Autodesk Fusion 360 part; units mm, degrees
(part 2 of 4)
  spline S394 degree 3 poles (77.092, 15.6185) (76.8084, 15.0287) (76.6767, 14.3737) (76.5494, 13.7318) knots 0 0 0 0 1 1 1 1
  spline S395 degree 3 poles (76.5494, 13.7318) (76.4799, 13.3813) (76.5996, 13.0055) (76.5054, 12.6609) knots 0 0 0 0 1 1 1 1
  spline S396 degree 3 poles (76.5054, 12.6609) (76.401, 12.2788) (76.1059, 11.9726) (75.9671, 11.6017) knots 0 0 0 0 1 1 1 1
  spline S397 degree 3 poles (75.9671, 11.6017) (75.8459, 11.2776) (75.8098, 10.9278) (75.7312, 10.5909) knots 0 0 0 0 1 1 1 1
  spline S398 degree 3 poles (77.2579, 14.4353) (77.0942, 14.4652) (76.9305, 14.4951) (76.7668, 14.525) knots 0 0 0 0 1 1 1 1
  spline S399 degree 3 poles (76.2224, 10.5718) (76.0243, 10.4293) (75.7374, 10.3626) (75.6282, 10.1444) knots 0 0 0 0 1 1 1 1
  spline S400 degree 3 poles (75.6282, 10.1444) (75.4268, 9.7418) (75.3959, 9.2709) (75.3477, 8.8234) knots 0 0 0 0 1 1 1 1
  spline S401 degree 3 poles (75.3477, 8.8234) (75.2928, 8.3128) (75.3293, 7.7964) (75.3201, 7.2829) knots 0 0 0 0 1 1 1 1
  spline S402 degree 3 poles (74.77, 0.2181) (74.6504, 0.8429) (74.4776, 1.4598) (74.4114, 2.0925) knots 0 0 0 0 1 1 1 1
  spline S403 degree 3 poles (74.4114, 2.0925) (74.3786, 2.4055) (74.3986, 2.7292) (74.4753, 3.0344) knots 0 0 0 0 1 1 1 1
  spline S404 degree 3 poles (74.4753, 3.0344) (74.5407, 3.2944) (74.7115, 3.5157) (74.8296, 3.7563) knots 0 0 0 0 1 1 1 1
  spline S405 degree 3 poles (74.4084, 0.1917) (74.5689, 0.7067) (74.7884, 1.2069) (74.89, 1.7368) knots 0 0 0 0 1 1 1 1
  spline S406 degree 3 poles (74.89, 1.7368) (74.9706, 2.1572) (74.9634, 2.5918) (74.9506, 3.0197) knots 0 0 0 0 1 1 1 1
  spline S407 degree 3 poles (74.9506, 3.0197) (74.9432, 3.2684) (74.8081, 3.5084) (74.8296, 3.7563) knots 0 0 0 0 1 1 1 1
  spline S408 degree 3 poles (74.8296, 3.7563) (74.9321, 4.9387) (75.0884, 6.1189) (75.3201, 7.2829) knots 0 0 0 0 1 1 1 1
  spline S409 degree 3 poles (75.3201, 7.2829) (75.4212, 7.7908) (75.6863, 8.2533) (75.8241, 8.7525) knots 0 0 0 0 1 1 1 1
  spline S410 degree 3 poles (75.8241, 8.7525) (76.047, 9.5598) (76.2121, 10.382) (76.4009, 11.1979) knots 0 0 0 0 1 1 1 1
  spline S411 degree 3 poles (76.4009, 11.1979) (76.444, 11.3845) (76.5062, 11.569) (76.5199, 11.76) knots 0 0 0 0 1 1 1 1
  spline S412 degree 3 poles (76.5199, 11.76) (76.5413, 12.0596) (76.4089, 12.3765) (76.5054, 12.6609) knots 0 0 0 0 1 1 1 1
  spline S413 degree 3 poles (76.5054, 12.6609) (76.6232, 13.0077) (76.9957, 13.2235) (77.1323, 13.5633) knots 0 0 0 0 1 1 1 1
  spline S414 degree 3 poles (77.1323, 13.5633) (77.2648, 13.8927) (77.1897, 14.2764) (77.2919, 14.6164) knots 0 0 0 0 1 1 1 1
  spline S415 degree 3 poles (77.2919, 14.6164) (77.6529, 15.8169) (78.1525, 16.9725) (78.5181, 18.1715) knots 0 0 0 0 1 1 1 1
  spline S416 degree 3 poles (78.5181, 18.1715) (78.7217, 18.8392) (78.8376, 19.5306) (78.9974, 20.2101) knots 0 0 0 0 1 1 1 1
  spline S417 degree 3 poles (79.9114, 55.8352) (80.0018, 55.3118) (80.1355, 54.7941) (80.1826, 54.2651) knots 0 0 0 0 1 1 1 1
  spline S418 degree 3 poles (80.1826, 54.2651) (80.2327, 53.7033) (80.2016, 53.1372) (80.2021, 52.5732) knots 0 0 0 0 1 1 1 1
  spline S419 degree 3 poles (80.2021, 52.5732) (80.2029, 51.5589) (80.2493, 50.5427) (80.1867, 49.5304) knots 0 0 0 0 1 1 1 1
  spline S420 degree 3 poles (80.1867, 49.5304) (80.1582, 49.0702) (80.0154, 48.6244) (79.9298, 48.1714) knots 0 0 0 0 1 1 1 1
  spline S421 degree 3 poles (79.8815, 67.9143) (79.9749, 67.5935) (80.1062, 67.2814) (80.1618, 66.952) knots 0 0 0 0 1 1 1 1
  spline S422 degree 3 poles (80.1618, 66.952) (80.206, 66.6894) (80.2356, 66.4133) (80.1783, 66.1533) knots 0 0 0 0 1 1 1 1
  spline S423 degree 3 poles (80.1783, 66.1533) (80.0552, 65.5942) (79.8112, 65.0687) (79.6277, 64.5264) knots 0 0 0 0 1 1 1 1
  spline S424 degree 3 poles (79.5785, 91.537) (79.7388, 91.1048) (79.9446, 90.6867) (80.0595, 90.2403) knots 0 0 0 0 1 1 1 1
  spline S425 degree 3 poles (80.0595, 90.2403) (80.1175, 90.0154) (80.0912, 89.7767) (80.0917, 89.5445) knots 0 0 0 0 1 1 1 1
  spline S426 degree 3 poles (80.0917, 89.5445) (80.1015, 84.6108) (80.0658, 79.677) (80.0904, 74.7433) knots 0 0 0 0 1 1 1 1
  spline S427 degree 3 poles (80.0904, 74.7433) (80.0948, 73.8732) (80.1608, 73.0044) (80.1787, 72.1345) knots 0 0 0 0 1 1 1 1
  spline S428 degree 3 poles (80.1787, 72.1345) (80.1839, 71.8819) (80.196, 71.6268) (80.1597, 71.3767) knots 0 0 0 0 1 1 1 1
  spline S429 degree 3 poles (80.1597, 71.3767) (80.0947, 70.9291) (79.9705, 70.4921) (79.8759, 70.0498) knots 0 0 0 0 1 1 1 1
  spline S430 degree 3 poles (79.0105, 108.9811) (79.3177, 108.5339) (79.6525, 108.1045) (79.932, 107.6395) knots 0 0 0 0 1 1 1 1
  spline S431 degree 3 poles (79.932, 107.6395) (79.967, 107.5812) (79.9385, 107.5036) (79.9392, 107.4356) knots 0 0 0 0 1 1 1 1
  spline S432 degree 3 poles (79.9392, 107.4356) (79.9902, 102.2627) (80.0602, 97.0898) (80.087, 91.9167) knots 0 0 0 0 1 1 1 1
  spline S433 degree 3 poles (80.087, 91.9167) (80.0884, 91.649) (80.0939, 91.3745) (80.0237, 91.1162) knots 0 0 0 0 1 1 1 1
  spline S434 degree 3 poles (80.0237, 91.1162) (79.9236, 90.7473) (79.7295, 90.4106) (79.5824, 90.0578) knots 0 0 0 0 1 1 1 1
  spline S435 degree 3 poles (81.6557, 96.4284) (81.1344, 96.4961) (80.6131, 96.5638) (80.0918, 96.6314) knots 0 0 0 0 1 1 1 1
  spline S436 degree 3 poles (126.938, 46.5861) (126.9859, 46.9193) (127.0338, 47.2526) (127.0817, 47.5858) knots 0 0 0 0 1 1 1 1
  spline S437 degree 3 poles (113.5695, 9.6089) (113.5669, 9.2811) (113.5643, 8.9533) (113.5617, 8.6255) knots 0 0 0 0 1 1 1 1
  spline S438 degree 3 poles (114.6587, 59.9943) (114.3579, 59.9988) (114.0571, 60.0032) (113.7562, 60.0077) knots 0 0 0 0 1 1 1 1
  spline S439 degree 3 poles (107.3619, 59.9943) (107.1224, 59.9938) (106.883, 59.9934) (106.6435, 59.9929) knots 0 0 0 0 1 1 1 1
  spline S440 degree 3 poles (91.5309, 60.5389) (91.4392, 60.798) (91.3475, 61.0572) (91.2558, 61.3163) knots 0 0 0 0 1 1 1 1
  spline S441 degree 3 poles (93.2706, 59.9738) (93.5427, 60.2052) (93.8147, 60.4367) (94.0867, 60.6681) knots 0 0 0 0 1 1 1 1
  spline S442 degree 3 poles (91.5309, 60.5389) (91.5604, 60.3114) (91.5898, 60.084) (91.6192, 59.8565) knots 0 0 0 0 1 1 1 1
  spline S443 degree 3 poles (122.187, 60.0082) (121.7808, 60.0892) (121.3824, 60.2359) (120.9686, 60.2512) knots 0 0 0 0 1 1 1 1
  spline S444 degree 3 poles (120.9686, 60.2512) (119.1221, 60.3194) (117.2722, 60.3165) (115.4253, 60.258) knots 0 0 0 0 1 1 1 1
  spline S445 degree 3 poles (115.4253, 60.258) (114.6969, 60.235) (113.9821, 60.0127) (113.2533, 60.0068) knots 0 0 0 0 1 1 1 1
  spline S446 degree 3 poles (113.2533, 60.0068) (113.021, 60.0049) (112.8268, 60.2232) (112.5948, 60.2352) knots 0 0 0 0 1 1 1 1
  spline S447 degree 3 poles (112.5948, 60.2352) (111.2245, 60.3059) (109.8505, 60.2555) (108.4784, 60.253) knots 0 0 0 0 1 1 1 1
  spline S448 degree 3 poles (108.4784, 60.253) (108.2642, 60.2526) (108.0473, 60.2639) (107.8365, 60.2264) knots 0 0 0 0 1 1 1 1
  spline S449 degree 3 poles (107.8365, 60.2264) (107.0992, 60.0953) (106.388, 59.8047) (105.6413, 59.7486) knots 0 0 0 0 1 1 1 1
  spline S450 degree 3 poles (105.6413, 59.7486) (104.2297, 59.6425) (102.8091, 59.6856) (101.3947, 59.7422) knots 0 0 0 0 1 1 1 1
  spline S451 degree 3 poles (101.3947, 59.7422) (100.8741, 59.763) (100.3692, 59.9384) (99.8499, 59.9804) knots 0 0 0 0 1 1 1 1
  spline S452 degree 3 poles (99.8499, 59.9804) (99.3911, 60.0175) (98.9282, 60.0105) (98.469, 59.979) knots 0 0 0 0 1 1 1 1
  spline S453 degree 3 poles (98.469, 59.979) (97.6609, 59.9234) (96.8629, 59.7272) (96.0529, 59.7195) knots 0 0 0 0 1 1 1 1
  spline S454 degree 3 poles (96.0529, 59.7195) (94.1791, 59.7015) (92.3077, 59.8681) (90.4341, 59.9021) knots 0 0 0 0 1 1 1 1
  spline S455 degree 3 poles (90.4341, 59.9021) (89.9009, 59.9117) (89.3666, 59.893) (88.835, 59.8501) knots 0 0 0 0 1 1 1 1
  spline S456 degree 3 poles (88.835, 59.8501) (88.6496, 59.8351) (88.4368, 59.8437) (88.2902, 59.7291) knots 0 0 0 0 1 1 1 1
  spline S457 degree 3 poles (88.2902, 59.7291) (87.9987, 59.5014) (87.7599, 59.1985) (87.5843, 58.873) knots 0 0 0 0 1 1 1 1
  spline S458 degree 3 poles (87.5843, 58.873) (87.5028, 58.7219) (87.5475, 58.5307) (87.5513, 58.3591) knots 0 0 0 0 1 1 1 1
  spline S459 degree 3 poles (87.5513, 58.3591) (87.5638, 57.7934) (87.5756, 57.2265) (87.6332, 56.6637) knots 0 0 0 0 1 1 1 1
  spline S460 degree 3 poles (87.6332, 56.6637) (87.6743, 56.2631) (87.8442, 55.8774) (87.8467, 55.4748) knots 0 0 0 0 1 1 1 1
  spline S461 degree 3 poles (87.8467, 55.4748) (87.8512, 54.7336) (87.6636, 54.0007) (87.6541, 53.2595) knots 0 0 0 0 1 1 1 1
  spline S462 degree 3 poles (87.6541, 53.2595) (87.6167, 50.3466) (87.6166, 47.432) (87.706, 44.5202) knots 0 0 0 0 1 1 1 1
  spline S463 degree 3 poles (87.706, 44.5202) (87.7152, 44.2221) (87.8678, 43.9461) (87.9487, 43.659) knots 0 0 0 0 1 1 1 1
  spline S464 degree 3 poles (87.9979, 36.6764) (87.9229, 36.2239) (87.7957, 35.7771) (87.7731, 35.319) knots 0 0 0 0 1 1 1 1
  spline S465 degree 3 poles (87.7731, 35.319) (87.7328, 34.5025) (87.759, 33.6828) (87.8097, 32.8668) knots 0 0 0 0 1 1 1 1
  spline S466 degree 3 poles (87.8097, 32.8668) (87.8225, 32.6602) (87.9116, 32.4654) (87.9626, 32.2647) knots 0 0 0 0 1 1 1 1
  spline S467 degree 3 poles (88.1957, 30.9055) (88.118, 31.3586) (87.9902, 31.8059) (87.9626, 32.2647) knots 0 0 0 0 1 1 1 1
  spline S468 degree 3 poles (87.9626, 32.2647) (87.933, 32.7581) (88.0043, 33.2525) (88.0251, 33.7463) knots 0 0 0 0 1 1 1 1
  spline S469 degree 3 poles (98.9943, 14.48) (99.0689, 14.5909) (99.1436, 14.7018) (99.2182, 14.8126) knots 0 0 0 0 1 1 1 1
  spline S470 degree 3 poles (102.6058, 5.998) (102.5228, 5.7723) (102.4398, 5.5466) (102.3568, 5.321) knots 0 0 0 0 1 1 1 1
  spline S471 degree 3 poles (88.0024, 59.4517) (88.0406, 58.5025) (88.154, 57.5534) (88.1169, 56.6042) knots 0 0 0 0 1 1 1 1
  spline S472 degree 3 poles (88.1169, 56.6042) (88.1017, 56.2174) (87.8475, 55.8619) (87.8467, 55.4748) knots 0 0 0 0 1 1 1 1
  spline S473 degree 3 poles (87.8467, 55.4748) (87.8454, 54.8647) (88.0854, 54.2733) (88.1106, 53.6637) knots 0 0 0 0 1 1 1 1
  spline S474 degree 3 poles (88.1106, 53.6637) (88.1921, 51.6938) (88.1601, 49.7208) (88.1662, 47.7493) knots 0 0 0 0 1 1 1 1
  spline S475 degree 3 poles (88.1662, 47.7493) (88.1694, 46.7375) (88.1922, 45.7245) (88.1385, 44.7142) knots 0 0 0 0 1 1 1 1
  spline S476 degree 3 poles (88.1385, 44.7142) (88.1195, 44.3573) (87.955, 44.0163) (87.9487, 43.659) knots 0 0 0 0 1 1 1 1
  spline S477 degree 3 poles (87.9487, 43.659) (87.908, 41.3317) (87.9056, 39.0021) (87.9979, 36.6764) knots 0 0 0 0 1 1 1 1
  spline S478 degree 3 poles (87.9979, 36.6764) (88.0141, 36.267) (88.2591, 35.8879) (88.2731, 35.4784) knots 0 0 0 0 1 1 1 1
  spline S479 degree 3 poles (88.2731, 35.4784) (88.3253, 33.9548) (88.1745, 32.4299) (88.1957, 30.9055) knots 0 0 0 0 1 1 1 1
  spline S480 degree 3 poles (88.1957, 30.9055) (88.199, 30.6714) (88.2691, 30.4406) (88.3461, 30.2195) knots 0 0 0 0 1 1 1 1
  spline S481 degree 3 poles (88.3461, 30.2195) (88.3895, 30.095) (88.4647, 29.9806) (88.5523, 29.8821) knots 0 0 0 0 1 1 1 1
  spline S482 degree 3 poles (88.5523, 29.8821) (89.1262, 29.2371) (89.7841, 28.6667) (90.3258, 27.9944) knots 0 0 0 0 1 1 1 1
  spline S483 degree 3 poles (90.3258, 27.9944) (90.6835, 27.5505) (90.8784, 26.9899) (91.2386, 26.548) knots 0 0 0 0 1 1 1 1
  spline S484 degree 3 poles (91.2386, 26.548) (91.6403, 26.0553) (92.1806, 25.6897) (92.5967, 25.2092) knots 0 0 0 0 1 1 1 1
  spline S485 degree 3 poles (92.5967, 25.2092) (93.3218, 24.3719) (93.9971, 23.4919) (94.656, 22.6017) knots 0 0 0 0 1 1 1 1
  spline S486 degree 3 poles (94.656, 22.6017) (94.7637, 22.4562) (94.7872, 22.2607) (94.8896, 22.1114) knots 0 0 0 0 1 1 1 1
  spline S487 degree 3 poles (94.8896, 22.1114) (95.0285, 21.9088) (95.2634, 21.7752) (95.3736, 21.5556) knots 0 0 0 0 1 1 1 1
  spline S488 degree 3 poles (95.3736, 21.5556) (95.4973, 21.3089) (95.4276, 20.987) (95.5717, 20.7516) knots 0 0 0 0 1 1 1 1
  spline S489 degree 3 poles (95.5717, 20.7516) (95.6351, 20.648) (95.8168, 20.7148) (95.9236, 20.6569) knots 0 0 0 0 1 1 1 1
  spline S490 degree 3 poles (95.9236, 20.6569) (96.0053, 20.6126) (96.0643, 20.5327) (96.1171, 20.4562) knots 0 0 0 0 1 1 1 1
  spline S491 degree 3 poles (96.1171, 20.4562) (96.5068, 19.8919) (96.912, 19.3356) (97.2487, 18.7382) knots 0 0 0 0 1 1 1 1
  spline S492 degree 3 poles (97.2487, 18.7382) (97.4861, 18.3172) (97.6108, 17.8403) (97.8334, 17.4113) knots 0 0 0 0 1 1 1 1
  spline S493 degree 3 poles (97.8334, 17.4113) (97.9225, 17.2396) (98.0923, 17.1181) (98.1791, 16.9452) knots 0 0 0 0 1 1 1 1
  spline S494 degree 3 poles (98.1791, 16.9452) (98.2599, 16.784) (98.2453, 16.5852) (98.3282, 16.425) knots 0 0 0 0 1 1 1 1
  spline S495 degree 3 poles (98.3282, 16.425) (98.5009, 16.0917) (98.7795, 15.8186) (98.9386, 15.4786) knots 0 0 0 0 1 1 1 1
  spline S496 degree 3 poles (98.9386, 15.4786) (99.5227, 14.2299) (100.0634, 12.9597) (100.5523, 11.6707) knots 0 0 0 0 1 1 1 1
  spline S497 degree 3 poles (100.5523, 11.6707) (100.7054, 11.2671) (100.7202, 10.8211) (100.8599, 10.4127) knots 0 0 0 0 1 1 1 1
  spline S498 degree 3 poles (100.8599, 10.4127) (100.9002, 10.295) (101.0423, 10.2318) (101.0847, 10.1149) knots 0 0 0 0 1 1 1 1
  spline S499 degree 3 poles (101.0847, 10.1149) (101.3358, 9.4211) (101.4896, 8.6949) (101.7336, 7.9986) knots 0 0 0 0 1 1 1 1
  spline S500 degree 3 poles (101.7336, 7.9986) (101.7697, 7.8955) (101.8986, 7.8364) (101.9205, 7.7294) knots 0 0 0 0 1 1 1 1
  spline S501 degree 3 poles (101.9205, 7.7294) (102.0347, 7.1735) (102.0196, 6.5961) (102.1356, 6.0406) knots 0 0 0 0 1 1 1 1
  spline S502 degree 3 poles (102.1356, 6.0406) (102.2157, 5.6568) (102.4342, 5.3097) (102.5062, 4.9243) knots 0 0 0 0 1 1 1 1
  spline S503 degree 3 poles (102.5062, 4.9243) (102.6128, 4.353) (102.5814, 3.7631) (102.6681, 3.1884) knots 0 0 0 0 1 1 1 1
  spline S504 degree 3 poles (102.6681, 3.1884) (102.7321, 2.7646) (102.8942, 2.3594) (102.9573, 1.9354) knots 0 0 0 0 1 1 1 1
  spline S505 degree 3 poles (102.9573, 1.9354) (103.0312, 1.4388) (102.9536, 0.9204) (103.0781, 0.4341) knots 0 0 0 0 1 1 1 1
  spline S506 degree 3 poles (103.0781, 0.4341) (103.1177, 0.2793) (103.3099, 0.2143) (103.4258, 0.1045) knots 0 0 0 0 1 1 1 1
  spline S507 degree 3 poles (100.304, 13.0648) (100.3455, 12.9599) (100.4087, 12.8611) (100.4285, 12.75) knots 0 0 0 0 1 1 1 1
  spline S508 degree 3 poles (100.4285, 12.75) (100.492, 12.3935) (100.511, 12.0305) (100.5523, 11.6707) knots 0 0 0 0 1 1 1 1
  spline S509 degree 3 poles (107.3619, 59.9943) (107.4569, 59.9303) (107.5409, 59.8457) (107.6469, 59.8023) knots 0 0 0 0 1 1 1 1
  spline S510 degree 3 poles (107.6469, 59.8023) (107.7416, 59.7635) (107.8477, 59.7551) (107.9501, 59.7534) knots 0 0 0 0 1 1 1 1
  spline S511 degree 3 poles (107.9501, 59.7534) (108.7435, 59.74) (109.5443, 59.6507) (110.3306, 59.757) knots 0 0 0 0 1 1 1 1
  spline S512 degree 3 poles (110.3306, 59.757) (110.7502, 59.8138) (111.1152, 60.0753) (111.5075, 60.2345) knots 0 0 0 0 1 1 1 1
  spline S513 degree 3 poles (111.0775, 59.9943) (111.2217, 59.9171) (111.351, 59.8005) (111.5101, 59.7628) knots 0 0 0 0 1 1 1 1
  spline S514 degree 3 poles (111.5101, 59.7628) (111.7171, 59.7138) (111.9352, 59.7361) (112.1478, 59.7409) knots 0 0 0 0 1 1 1 1
  spline S515 degree 3 poles (112.1478, 59.7409) (112.3352, 59.7451) (112.5257, 59.7459) (112.7079, 59.7897) knots 0 0 0 0 1 1 1 1
  spline S516 degree 3 poles (112.7079, 59.7897) (112.8981, 59.8354) (113.0715, 59.9344) (113.2533, 60.0068) knots 0 0 0 0 1 1 1 1
  spline S517 degree 3 poles (116.549, 60.2371) (116.549, 60.0825) (116.549, 59.9279) (116.549, 59.7733) knots 0 0 0 0 1 1 1 1
  spline S518 degree 3 poles (114.6587, 59.9943) (114.7193, 59.9458) (114.7678, 59.8764) (114.8403, 59.8488) knots 0 0 0 0 1 1 1 1
  spline S519 degree 3 poles (114.8403, 59.8488) (114.9866, 59.7932) (115.143, 59.7553) (115.2994, 59.7506) knots 0 0 0 0 1 1 1 1
  spline S520 degree 3 poles (115.2994, 59.7506) (116.1894, 59.7241) (117.0862, 59.6525) (117.9707, 59.7555) knots 0 0 0 0 1 1 1 1
  spline S521 degree 3 poles (117.9707, 59.7555) (118.5044, 59.8177) (118.9955, 60.0791) (119.508, 60.2409) knots 0 0 0 0 1 1 1 1
  spline S522 degree 3 poles (113.5695, 9.6089) (113.6706, 9.9448) (113.7371, 10.2932) (113.8727, 10.6167) knots 0 0 0 0 1 1 1 1
  spline S523 degree 3 poles (113.8727, 10.6167) (114.1011, 11.1616) (114.423, 11.6637) (114.6579, 12.2058) knots 0 0 0 0 1 1 1 1
  spline S524 degree 3 poles (114.6579, 12.2058) (115.2453, 13.5615) (115.7231, 14.9641) (116.3383, 16.3075) knots 0 0 0 0 1 1 1 1
  spline S525 degree 3 poles (116.3383, 16.3075) (116.8236, 17.3673) (117.3871, 18.3904) (117.956, 19.4079) knots 0 0 0 0 1 1 1 1
  spline S526 degree 3 poles (117.956, 19.4079) (118.3649, 20.1393) (118.8074, 20.8524) (119.27, 21.551) knots 0 0 0 0 1 1 1 1
  spline S527 degree 3 poles (119.27, 21.551) (119.8502, 22.4271) (120.4527, 23.289) (121.0829, 24.1299) knots 0 0 0 0 1 1 1 1
  spline S528 degree 3 poles (121.0829, 24.1299) (121.7231, 24.9842) (122.4041, 25.8073) (123.0793, 26.6343) knots 0 0 0 0 1 1 1 1
  spline S529 degree 3 poles (123.0793, 26.6343) (123.1955, 26.7765) (123.3149, 26.9189) (123.4561, 27.0364) knots 0 0 0 0 1 1 1 1
  spline S530 degree 3 poles (123.4561, 27.0364) (123.7043, 27.2428) (124.0151, 27.3727) (124.2425, 27.6019) knots 0 0 0 0 1 1 1 1
  spline S531 degree 3 poles (124.2425, 27.6019) (124.8517, 28.2158) (125.3548, 28.9282) (125.9531, 29.5526) knots 0 0 0 0 1 1 1 1
  spline S532 degree 3 poles (125.9531, 29.5526) (126.3072, 29.9222) (126.9547, 30.0868) (127.095, 30.579) knots 0 0 0 0 1 1 1 1
  spline S533 degree 3 poles (127.095, 30.579) (127.3887, 31.6098) (127.2323, 32.7244) (127.1618, 33.7939) knots 0 0 0 0 1 1 1 1
  spline S534 degree 3 poles (127.1618, 33.7939) (127.1295, 34.2845) (126.8815, 35.7038) (126.789, 35.2209) knots 0 0 0 0 1 1 1 1
  spline S535 degree 3 poles (126.789, 35.2209) (126.5274, 33.8548) (126.724, 32.439) (126.6364, 31.0508) knots 0 0 0 0 1 1 1 1
  spline S536 degree 3 poles (126.6364, 31.0508) (126.6203, 30.794) (126.5851, 30.5294) (126.4783, 30.2953) knots 0 0 0 0 1 1 1 1
  spline S537 degree 3 poles (126.4783, 30.2953) (126.3525, 30.0195) (126.1282, 29.8002) (125.9531, 29.5526) knots 0 0 0 0 1 1 1 1
  spline S538 degree 3 poles (126.9452, 33.7354) (126.8662, 34.5258) (126.728, 35.3126) (126.7084, 36.1067) knots 0 0 0 0 1 1 1 1
  spline S539 degree 3 poles (126.7084, 36.1067) (126.6364, 39.0193) (126.7052, 41.9337) (126.6707, 44.847) knots 0 0 0 0 1 1 1 1
  spline S540 degree 3 poles (126.6707, 44.847) (126.6701, 44.8973) (126.6468, 44.9571) (126.6031, 44.982) knots 0 0 0 0 1 1 1 1
  spline S541 degree 3 poles (126.6031, 44.982) (126.3028, 45.1529) (125.9177, 45.1858) (125.6637, 45.4201) knots 0 0 0 0 1 1 1 1
  spline S542 degree 3 poles (125.6637, 45.4201) (125.5225, 45.5504) (125.5695, 45.7927) (125.5224, 45.979) knots 0 0 0 0 1 1 1 1
  spline S543 degree 3 poles (112.2476, 0.2003) (112.2429, 0.55) (112.2383, 0.8998) (112.2336, 1.2495) knots 0 0 0 0 1 1 1 1
  spline S544 degree 3 poles (114.6579, 12.2058) (114.5509, 11.6204) (114.4655, 11.0306) (114.3369, 10.4496) knots 0 0 0 0 1 1 1 1
  spline S545 degree 3 poles (114.3369, 10.4496) (114.2803, 10.1938) (114.2057, 9.9403) (114.1032, 9.6991) knots 0 0 0 0 1 1 1 1
  spline S546 degree 3 poles (114.1032, 9.6991) (113.9464, 9.3302) (113.6948, 9.0036) (113.5617, 8.6255) knots 0 0 0 0 1 1 1 1
  spline S547 degree 3 poles (113.5617, 8.6255) (113.391, 8.1404) (113.305, 7.6292) (113.1979, 7.1261) knots 0 0 0 0 1 1 1 1
  spline S548 degree 3 poles (113.1979, 7.1261) (113.0157, 6.2707) (112.8357, 5.4142) (112.6941, 4.5511) knots 0 0 0 0 1 1 1 1
  spline S549 degree 3 poles (112.6941, 4.5511) (112.5141, 3.4546) (112.4386, 2.3416) (112.2336, 1.2495) knots 0 0 0 0 1 1 1 1
  spline S550 degree 3 poles (112.2336, 1.2495) (112.1603, 0.8587) (111.9857, 0.4939) (111.8617, 0.1161) knots 0 0 0 0 1 1 1 1
  spline S551 degree 3 poles (126.5749, 45.0025) (126.6297, 47.3002) (126.716, 49.5973) (126.7395, 51.8956) knots 0 0 0 0 1 1 1 1
  spline S552 degree 3 poles (126.7395, 51.8956) (126.7423, 52.1713) (126.6378, 52.443) (126.6537, 52.7182) knots 0 0 0 0 1 1 1 1
  spline S553 degree 3 poles (126.6537, 52.7182) (126.685, 53.2575) (126.8689, 53.7828) (126.8801, 54.3228) knots 0 0 0 0 1 1 1 1
  spline S554 degree 3 poles (126.8801, 54.3228) (126.9183, 56.1585) (126.8278, 57.9946) (126.8017, 59.8305) knots 0 0 0 0 1 1 1 1
  spline S555 degree 3 poles (127.1559, 52.127) (127.1081, 52.0588) (127.0881, 51.9572) (127.0124, 51.9224) knots 0 0 0 0 1 1 1 1
  spline S556 degree 3 poles (127.0124, 51.9224) (126.9306, 51.8847) (126.8324, 51.9318) (126.7424, 51.9365) knots 0 0 0 0 1 1 1 1
  spline S557 degree 3 poles (126.9475, 48.3983) (126.9922, 48.1275) (127.0369, 47.8566) (127.0817, 47.5858) knots 0 0 0 0 1 1 1 1
  spline S558 degree 3 poles (127.2479, 35.1262) (127.1925, 39.2794) (127.1041, 43.4323) (127.0817, 47.5858) knots 0 0 0 0 1 1 1 1
  spline S559 degree 3 poles (127.0817, 47.5858) (127.0793, 48.023) (127.1654, 48.457) (127.1735, 48.8941) knots 0 0 0 0 1 1 1 1
  spline S560 degree 3 poles (127.1735, 48.8941) (127.1966, 50.1308) (127.1821, 51.368) (127.1754, 52.605) knots 0 0 0 0 1 1 1 1
  spline S561 degree 3 poles (127.1754, 52.605) (127.1741, 52.8394) (127.1894, 53.0767) (127.1497, 53.3077) knots 0 0 0 0 1 1 1 1
  spline S562 degree 3 poles (127.1497, 53.3077) (127.0904, 53.6528) (126.97, 53.9844) (126.8801, 54.3228) knots 0 0 0 0 1 1 1 1
  spline S563 degree 3 poles (132.1879, 57.8221) (130.5903, 58.4578) (129.0308, 59.1992) (127.3952, 59.7294) knots 0 0 0 0 1 1 1 1
  spline S564 degree 3 poles (127.3952, 59.7294) (126.8222, 59.9152) (126.204, 59.9247) (125.6026, 59.9569) knots 0 0 0 0 1 1 1 1
  spline S565 degree 3 poles (125.6026, 59.9569) (124.4655, 60.0177) (123.3246, 60.0568) (122.187, 60.0082) knots 0 0 0 0 1 1 1 1
  spline S566 degree 3 poles (122.187, 60.0082) (121.8248, 59.9927) (121.488, 59.7981) (121.127, 59.7658) knots 0 0 0 0 1 1 1 1
  spline S567 degree 3 poles (121.127, 59.7658) (120.5876, 59.7175) (120.0408, 59.7092) (119.5024, 59.7679) knots 0 0 0 0 1 1 1 1
  spline S568 degree 3 poles (119.5024, 59.7679) (119.3288, 59.7868) (119.1874, 59.9188) (119.0299, 59.9943) knots 0 0 0 0 1 1 1 1
  spline S569 degree 3 poles (106.6435, 59.9929) (106.3094, 60.0741) (105.9841, 60.2136) (105.641, 60.2365) knots 0 0 0 0 1 1 1 1
  spline S570 degree 3 poles (105.641, 60.2365) (104.6812, 60.3006) (103.7172, 60.2592) (102.7554, 60.2525) knots 0 0 0 0 1 1 1 1
  spline S571 degree 3 poles (102.7554, 60.2525) (102.1731, 60.2484) (101.5874, 60.2742) (101.0093, 60.2044) knots 0 0 0 0 1 1 1 1
  spline S572 degree 3 poles (101.0093, 60.2044) (100.8629, 60.1866) (100.7647, 60.0222) (100.6199, 59.9943) knots 0 0 0 0 1 1 1 1
  spline S573 degree 3 poles (100.6199, 59.9943) (100.3678, 59.9456) (100.1066, 59.985) (99.8499, 59.9804) knots 0 0 0 0 1 1 1 1
  spline S574 degree 3 poles (97.4441, 60.6665) (97.4568, 60.4831) (97.4694, 60.2996) (97.4821, 60.1162) knots 0 0 0 0 1 1 1 1
  spline S575 degree 3 poles (91.2558, 61.3163) (91.7612, 61.2238) (92.273, 61.1615) (92.7719, 61.0386) knots 0 0 0 0 1 1 1 1
  spline S576 degree 3 poles (92.7719, 61.0386) (93.6293, 60.8274) (94.4614, 60.52) (95.3203, 60.3151) knots 0 0 0 0 1 1 1 1
  spline S577 degree 3 poles (95.3203, 60.3151) (95.5364, 60.2636) (95.7641, 60.2529) (95.9854, 60.2723) knots 0 0 0 0 1 1 1 1
  spline S578 degree 3 poles (95.9854, 60.2723) (96.1437, 60.2861) (96.2821, 60.4107) (96.4411, 60.413) knots 0 0 0 0 1 1 1 1
  spline S579 degree 3 poles (96.4411, 60.413) (96.5406, 60.4144) (96.6123, 60.3033) (96.7097, 60.2825) knots 0 0 0 0 1 1 1 1
  spline S580 degree 3 poles (96.7097, 60.2825) (97.2916, 60.1579) (97.8826, 60.0801) (98.469, 59.979) knots 0 0 0 0 1 1 1 1
  spline S581 degree 3 poles (127.286, 34.8589) (127.2733, 34.948) (127.2606, 35.0371) (127.2479, 35.1262) knots 0 0 0 0 1 1 1 1
  spline S582 degree 3 poles (95.4605, 92.5559) (95.3904, 92.4042) (95.3202, 92.2526) (95.25, 92.1009) knots 0 0 0 0 1 1 1 1
  spline S583 degree 3 poles (98.1279, 23.583) (98.0091, 23.6961) (97.8903, 23.8092) (97.7715, 23.9223) knots 0 0 0 0 1 1 1 1
  spline S584 degree 3 poles (118.9919, 100.9952) (118.977, 101.2153) (118.9621, 101.4355) (118.9472, 101.6557) knots 0 0 0 0 1 1 1 1
  spline S585 degree 3 poles (126.9225, 39.9955) (126.9225, 39.261) (126.9225, 38.5265) (126.9225, 37.792) knots 0 0 0 0 1 1 1 1
  spline S586 degree 3 poles (128.0742, 83.7969) (128.0973, 83.8414) (128.1205, 83.8859) (128.1436, 83.9304) knots 0 0 0 0 1 1 1 1
  spline S587 degree 3 poles (147.4067, 52.5952) (147.4384, 52.1666) (147.4701, 51.738) (147.5018, 51.3094) knots 0 0 0 0 1 1 1 1
  spline S588 degree 3 poles (136.9862, 37.5786) (137.0701, 38.0642) (137.1539, 38.5497) (137.2378, 39.0352) knots 0 0 0 0 1 1 1 1
  spline S589 degree 3 poles (137.2443, 43.6547) (137.1597, 43.1481) (136.9912, 42.6485) (136.9905, 42.1349) knots 0 0 0 0 1 1 1 1
  spline S590 degree 3 poles (136.9905, 42.1349) (136.9898, 41.6459) (137.2012, 41.1768) (137.2401, 40.6893) knots 0 0 0 0 1 1 1 1
  spline S591 degree 3 poles (137.2401, 40.6893) (137.284, 40.1397) (137.1942, 39.5848) (137.2378, 39.0352) knots 0 0 0 0 1 1 1 1
  spline S592 degree 3 poles (137.2378, 39.0352) (137.2815, 38.4845) (137.4491, 37.949) (137.5012, 37.3991) knots 0 0 0 0 1 1 1 1
  spline S593 degree 3 poles (137.5012, 37.3991) (137.5267, 37.1299) (137.5169, 36.8547) (137.4696, 36.5885) knots 0 0 0 0 1 1 1 1
  spline S594 degree 3 poles (137.4696, 36.5885) (137.4267, 36.3465) (137.312, 36.1229) (137.2332, 35.8901) knots 0 0 0 0 1 1 1 1
  spline S595 degree 3 poles (136.9993, 0.0952) (137.0193, 1.047) (136.999, 2.0005) (137.0593, 2.9506) knots 0 0 0 0 1 1 1 1
  spline S596 degree 3 poles (137.0593, 2.9506) (137.0755, 3.2055) (137.2268, 3.4426) (137.2282, 3.698) knots 0 0 0 0 1 1 1 1
  spline S597 degree 3 poles (137.2282, 3.698) (137.2848, 14.4285) (137.3108, 25.1597) (137.2332, 35.8901) knots 0 0 0 0 1 1 1 1
  spline S598 degree 3 poles (137.2332, 35.8901) (137.2314, 36.1391) (137.0245, 36.3498) (136.9902, 36.5964) knots 0 0 0 0 1 1 1 1
  spline S599 degree 3 poles (136.9902, 36.5964) (136.972, 36.7276) (137.0818, 36.8508) (137.0812, 36.9832) knots 0 0 0 0 1 1 1 1
  spline S600 degree 3 poles (137.0812, 36.9832) (137.0804, 37.1842) (137.0179, 37.3802) (136.9862, 37.5786) knots 0 0 0 0 1 1 1 1
  spline S601 degree 3 poles (137.4733, 0.1324) (137.467, 1.104) (137.5211, 2.0778) (137.4544, 3.0471) knots 0 0 0 0 1 1 1 1
  spline S602 degree 3 poles (137.4544, 3.0471) (137.4387, 3.2763) (137.3036, 3.481) (137.2282, 3.698) knots 0 0 0 0 1 1 1 1
  spline S603 degree 3 poles (137.2401, 40.6893) (137.3201, 41.0087) (137.4292, 41.3222) (137.48, 41.6475) knots 0 0 0 0 1 1 1 1
  spline S604 degree 3 poles (137.48, 41.6475) (137.5167, 41.8824) (137.5291, 42.1243) (137.5014, 42.3604) knots 0 0 0 0 1 1 1 1
  spline S605 degree 3 poles (137.5014, 42.3604) (137.45, 42.7973) (137.2704, 43.2156) (137.2443, 43.6547) knots 0 0 0 0 1 1 1 1
  spline S606 degree 3 poles (137.2443, 43.6547) (137.1857, 44.6369) (137.3012, 45.624) (137.2483, 46.6065) knots 0 0 0 0 1 1 1 1
  spline S607 degree 3 poles (137.2483, 46.6065) (137.2249, 47.0408) (137.0468, 47.4566) (137.016, 47.8904) knots 0 0 0 0 1 1 1 1
  spline S608 degree 3 poles (137.016, 47.8904) (136.9521, 48.7924) (136.9626, 49.6984) (136.9652, 50.6027) knots 0 0 0 0 1 1 1 1
  spline S609 degree 3 poles (136.9652, 50.6027) (136.9759, 54.312) (137.0512, 58.0211) (137.0561, 61.7304) knots 0 0 0 0 1 1 1 1
  spline S610 degree 3 poles (137.0561, 61.7304) (137.0693, 71.8786) (137.0145, 82.0267) (137.0194, 92.1749) knots 0 0 0 0 1 1 1 1
  spline S611 degree 3 poles (137.0194, 92.1749) (137.0207, 94.8012) (136.9811, 97.4291) (137.0748, 100.0538) knots 0 0 0 0 1 1 1 1
  spline S612 degree 3 poles (137.0748, 100.0538) (137.0966, 100.6668) (137.2685, 101.2652) (137.3654, 101.871) knots 0 0 0 0 1 1 1 1
  spline S613 degree 3 poles (137.2221, 50.2047) (137.3171, 49.5794) (137.5023, 48.9612) (137.5069, 48.3287) knots 0 0 0 0 1 1 1 1
  spline S614 degree 3 poles (137.5069, 48.3287) (137.5111, 47.7482) (137.3345, 47.1806) (137.2483, 46.6065) knots 0 0 0 0 1 1 1 1
  spline S615 degree 3 poles (147.4179, 94.1208) (147.3396, 93.7504) (147.2353, 93.3845) (147.1831, 93.0096) knots 0 0 0 0 1 1 1 1
  spline S616 degree 3 poles (147.1831, 93.0096) (147.1523, 92.7881) (147.1696, 92.5625) (147.1698, 92.339) knots 0 0 0 0 1 1 1 1
  spline S617 degree 3 poles (147.1698, 92.339) (147.1767, 83.114) (147.1839, 73.889) (147.2045, 64.664) knots 0 0 0 0 1 1 1 1
  spline S618 degree 3 poles (147.2045, 64.664) (147.2137, 60.5605) (147.1677, 56.4561) (147.2591, 52.3536) knots 0 0 0 0 1 1 1 1
  spline S619 degree 3 poles (147.2591, 52.3536) (147.267, 51.9964) (147.4209, 51.6575) (147.5018, 51.3094) knots 0 0 0 0 1 1 1 1
  spline S620 degree 3 poles (147.503, 50.7547) (147.4119, 50.3886) (147.2489, 50.0332) (147.2296, 49.6564) knots 0 0 0 0 1 1 1 1
  spline S621 degree 3 poles (147.2296, 49.6564) (147.1839, 48.7648) (147.2829, 47.8717) (147.3096, 46.9794) knots 0 0 0 0 1 1 1 1
  spline S622 degree 3 poles (145.171, 102.6184) (145.6273, 102.9689) (146.058, 103.3555) (146.5399, 103.6698) knots 0 0 0 0 1 1 1 1
  spline S623 degree 3 poles (146.5399, 103.6698) (146.6229, 103.7239) (146.7377, 103.7212) (146.8353, 103.7039) knots 0 0 0 0 1 1 1 1
  spline S624 degree 3 poles (146.8353, 103.7039) (146.9187, 103.6891) (147.0108, 103.6498) (147.0565, 103.5783) knots 0 0 0 0 1 1 1 1
  spline S625 degree 3 poles (147.0565, 103.5783) (147.1673, 103.4047) (147.2727, 103.209) (147.2826, 103.0033) knots 0 0 0 0 1 1 1 1
  spline S626 degree 3 poles (147.2826, 103.0033) (147.3129, 102.3716) (147.1847, 101.7414) (147.175, 101.1091) knots 0 0 0 0 1 1 1 1
  spline S627 degree 3 poles (147.175, 101.1091) (147.1506, 99.518) (147.1168, 97.9252) (147.1803, 96.3352) knots 0 0 0 0 1 1 1 1
  spline S628 degree 3 poles (147.1803, 96.3352) (147.1974, 95.9077) (147.3705, 95.499) (147.4161, 95.0737) knots 0 0 0 0 1 1 1 1
  spline S629 degree 3 poles (147.4161, 95.0737) (147.45, 94.7578) (147.3781, 94.4359) (147.4179, 94.1208) knots 0 0 0 0 1 1 1 1
  spline S630 degree 3 poles (147.4179, 94.1208) (147.4651, 93.7463) (147.6149, 93.3906) (147.6754, 93.0181) knots 0 0 0 0 1 1 1 1
  spline S631 degree 3 poles (147.6754, 93.0181) (147.7058, 92.8309) (147.6892, 92.6389) (147.6893, 92.4493) knots 0 0 0 0 1 1 1 1
  spline S632 degree 3 poles (147.6893, 92.4493) (147.6966, 80.0536) (147.7006, 67.6579) (147.6975, 55.2623) knots 0 0 0 0 1 1 1 1
  spline S633 degree 3 poles (147.6975, 55.2623) (147.6974, 54.5574) (147.7144, 53.8518) (147.6796, 53.1478) knots 0 0 0 0 1 1 1 1
  spline S634 degree 3 poles (147.6796, 53.1478) (147.6491, 52.5329) (147.4975, 51.925) (147.5018, 51.3094) knots 0 0 0 0 1 1 1 1
  spline S635 degree 3 poles (147.5018, 51.3094) (147.5069, 50.5998) (147.7393, 49.8994) (147.7078, 49.1905) knots 0 0 0 0 1 1 1 1
  spline S636 degree 3 poles (147.7078, 49.1905) (147.6746, 48.4424) (147.4043, 47.7223) (147.3096, 46.9794) knots 0 0 0 0 1 1 1 1
  spline S637 degree 3 poles (147.3096, 46.9794) (147.2646, 46.6261) (147.2849, 46.2672) (147.2898, 45.911) knots 0 0 0 0 1 1 1 1
  spline S638 degree 3 poles (147.2898, 45.911) (147.3196, 43.7464) (147.4074, 41.5825) (147.4138, 39.4177) knots 0 0 0 0 1 1 1 1
  spline S639 degree 3 poles (147.4138, 39.4177) (147.4157, 38.7527) (147.3214, 38.0902) (147.3147, 37.4253) knots 0 0 0 0 1 1 1 1
  spline S640 degree 3 poles (147.3147, 37.4253) (147.2858, 34.5672) (147.2424, 31.7081) (147.307, 28.8506) knots 0 0 0 0 1 1 1 1
  spline S641 degree 3 poles (147.307, 28.8506) (147.3231, 28.1411) (147.4965, 27.4433) (147.5566, 26.7361) knots 0 0 0 0 1 1 1 1
  spline S642 degree 3 poles (147.5566, 26.7361) (147.5805, 26.4539) (147.5862, 26.1683) (147.5587, 25.8864) knots 0 0 0 0 1 1 1 1
  spline S643 degree 3 poles (147.5587, 25.8864) (147.5125, 25.4144) (147.3881, 24.9525) (147.336, 24.4811) knots 0 0 0 0 1 1 1 1
  spline S644 degree 3 poles (147.336, 24.4811) (147.311, 24.2547) (147.3276, 24.0256) (147.3278, 23.7978) knots 0 0 0 0 1 1 1 1
  spline S645 degree 3 poles (147.3278, 23.7978) (147.3345, 17.724) (147.3472, 11.6501) (147.3568, 5.5763) knots 0 0 0 0 1 1 1 1
  spline S646 degree 3 poles (147.5568, 36.779) (147.509, 37.5335) (147.4612, 38.2881) (147.4134, 39.0426) knots 0 0 0 0 1 1 1 1
  spline S647 degree 3 poles (147.4404, 32.0087) (147.3994, 31.7966) (147.3584, 31.5846) (147.3174, 31.3725) knots 0 0 0 0 1 1 1 1
  spline S648 degree 3 poles (147.5857, 33.0628) (147.4983, 33.0874) (147.4109, 33.112) (147.3235, 33.1366) knots 0 0 0 0 1 1 1 1
  spline S649 degree 3 poles (147.3277, 1.6859) (147.3299, 2.8217) (147.2941, 3.9582) (147.3342, 5.0932) knots 0 0 0 0 1 1 1 1
  spline S650 degree 3 poles (147.3342, 5.0932) (147.3717, 6.1536) (146.5303, 8.0139) (147.5604, 8.2682) knots 0 0 0 0 1 1 1 1
  spline S651 degree 3 poles (147.5604, 8.2682) (148.5506, 8.5127) (147.8304, 6.2427) (147.8608, 5.2232) knots 0 0 0 0 1 1 1 1
  spline S652 degree 3 poles (147.8608, 5.2232) (147.8902, 4.2388) (147.7463, 3.2559) (147.7394, 2.271) knots 0 0 0 0 1 1 1 1
  spline S653 degree 3 poles (147.7394, 2.271) (147.7384, 2.1306) (147.8314, 2.0016) (147.8371, 1.8613) knots 0 0 0 0 1 1 1 1
  spline S654 degree 3 poles (147.8371, 1.8613) (147.8576, 1.3509) (147.8241, 0.8397) (147.8175, 0.3289) knots 0 0 0 0 1 1 1 1
  spline S655 degree 3 poles (147.5587, 25.8864) (147.6343, 25.5632) (147.7422, 25.246) (147.7857, 24.917) knots 0 0 0 0 1 1 1 1
  spline S656 degree 3 poles (147.7857, 24.917) (147.8247, 24.6223) (147.8042, 24.3226) (147.8049, 24.0253) knots 0 0 0 0 1 1 1 1
  spline S657 degree 3 poles (147.8049, 24.0253) (147.8208, 17.8811) (147.8253, 11.737) (147.8355, 5.5929) knots 0 0 0 0 1 1 1 1
  spline S658 degree 3 poles (147.6052, 48.9137) (147.6668, 47.8588) (147.7785, 46.8055) (147.79, 45.7488) knots 0 0 0 0 1 1 1 1
  spline S659 degree 3 poles (147.79, 45.7488) (147.8489, 40.3494) (147.8126, 34.9494) (147.8165, 29.5497) knots 0 0 0 0 1 1 1 1
  spline S660 degree 3 poles (147.8165, 29.5497) (147.8168, 29.1792) (147.8367, 28.8071) (147.8027, 28.4382) knots 0 0 0 0 1 1 1 1
  spline S661 degree 3 poles (147.8027, 28.4382) (147.7499, 27.8673) (147.6386, 27.3035) (147.5566, 26.7361) knots 0 0 0 0 1 1 1 1
  spline S662 degree 3 poles (147.4161, 95.0737) (147.503, 95.5447) (147.651, 96.0085) (147.6769, 96.4869) knots 0 0 0 0 1 1 1 1
  spline S663 degree 3 poles (147.6769, 96.4869) (147.759, 98.0058) (147.5653, 99.5388) (147.7394, 101.05) knots 0 0 0 0 1 1 1 1
  spline S664 degree 3 poles (147.7394, 101.05) (147.7595, 101.2249) (148.0801, 101.1567) (148.2262, 101.255) knots 0 0 0 0 1 1 1 1
  spline S665 degree 3 poles (148.2262, 101.255) (148.2952, 101.3015) (148.3993, 101.3941) (148.3587, 101.4667) knots 0 0 0 0 1 1 1 1
  spline S666 degree 3 poles (148.3587, 101.4667) (148.267, 101.6304) (148.0891, 101.7437) (147.9144, 101.8119) knots 0 0 0 0 1 1 1 1
  spline S667 degree 3 poles (147.9144, 101.8119) (147.3106, 102.0479) (146.6945, 102.2912) (146.0509, 102.3686) knots 0 0 0 0 1 1 1 1
  spline S668 degree 3 poles (146.0509, 102.3686) (145.1366, 102.4785) (144.2058, 102.2904) (143.2882, 102.3681) knots 0 0 0 0 1 1 1 1
  spline S669 degree 3 poles (143.2882, 102.3681) (142.4228, 102.4413) (141.5878, 102.7495) (140.7221, 102.8195) knots 0 0 0 0 1 1 1 1
  spline S670 degree 3 poles (140.7221, 102.8195) (139.8241, 102.8922) (138.9181, 102.8586) (138.0194, 102.7945) knots 0 0 0 0 1 1 1 1
  spline S671 degree 3 poles (138.0194, 102.7945) (137.8445, 102.7821) (137.6351, 102.7353) (137.5338, 102.5922) knots 0 0 0 0 1 1 1 1
  spline S672 degree 3 poles (137.5338, 102.5922) (137.3911, 102.3907) (137.3661, 102.1178) (137.3654, 101.871) knots 0 0 0 0 1 1 1 1
  spline S673 degree 3 poles (137.3654, 101.871) (137.362, 100.8411) (137.5162, 99.8153) (137.5216, 98.7855) knots 0 0 0 0 1 1 1 1
  spline S674 degree 3 poles (137.5216, 98.7855) (137.5638, 90.6839) (137.5897, 82.5817) (137.508, 74.4804) knots 0 0 0 0 1 1 1 1
  spline S675 degree 3 poles (137.508, 74.4804) (137.4975, 73.4415) (137.3328, 72.41) (137.2452, 71.3748) knots 0 0 0 0 1 1 1 1
  spline S676 degree 3 poles (142.8687, 102.5922) (143.0097, 102.6624) (143.1354, 102.7828) (143.2916, 102.8029) knots 0 0 0 0 1 1 1 1
  spline S677 degree 3 poles (143.2916, 102.8029) (143.6939, 102.8545) (144.1091, 102.8739) (144.5084, 102.8025) knots 0 0 0 0 1 1 1 1
  spline S678 degree 3 poles (144.5084, 102.8025) (144.8859, 102.7349) (145.2252, 102.5292) (145.5836, 102.3926) knots 0 0 0 0 1 1 1 1
  spline S679 degree 3 poles (137.4625, 102.3728) (139.4044, 102.3712) (141.3463, 102.3696) (143.2882, 102.3681) knots 0 0 0 0 1 1 1 1
  spline S680 degree 3 poles (137.2546, 78.6208) (137.3311, 78.2894) (137.4076, 77.9579) (137.4841, 77.6265) knots 0 0 0 0 1 1 1 1
  spline S681 degree 3 poles (137.2546, 77.748) (137.3284, 78.237) (137.4023, 78.726) (137.4761, 79.2149) knots 0 0 0 0 1 1 1 1
  spline S682 degree 3 poles (137.4513, 66.9197) (137.467, 68.1388) (137.5084, 69.3579) (137.4983, 70.577) knots 0 0 0 0 1 1 1 1
  spline S683 degree 3 poles (137.4983, 70.577) (137.4913, 71.4217) (137.4329, 72.2652) (137.4002, 73.1093) knots 0 0 0 0 1 1 1 1
  spline S684 degree 3 poles (137.2434, 67.5157) (137.3128, 67.317) (137.4156, 67.1271) (137.4513, 66.9197) knots 0 0 0 0 1 1 1 1
  spline S685 degree 3 poles (137.4513, 66.9197) (137.5021, 66.6251) (137.4998, 66.323) (137.5004, 66.024) knots 0 0 0 0 1 1 1 1
  spline S686 degree 3 poles (137.5004, 66.024) (137.5104, 60.2963) (137.4888, 54.5687) (137.483, 48.841) knots 0 0 0 0 1 1 1 1
  spline S687 degree 3 poles (152.7785, 117.5718) (152.8678, 117.9626) (152.9572, 118.3534) (153.0465, 118.7443) knots 0 0 0 0 1 1 1 1
  spline S688 degree 3 poles (161.9459, 165.2984) (161.6838, 165.2748) (161.4217, 165.2513) (161.1596, 165.2277) knots 0 0 0 0 1 1 1 1
  spline S689 degree 3 poles (175.4375, 165.4307) (175.1951, 165.4175) (174.9527, 165.4042) (174.7102, 165.391) knots 0 0 0 0 1 1 1 1
  spline S690 degree 3 poles (179.6496, 155.1791) (179.4867, 155.5492) (179.3238, 155.9192) (179.1608, 156.2893) knots 0 0 0 0 1 1 1 1
  spline S691 degree 3 poles (171.9272, 0.2531) (172.0962, 0.7922) (172.2652, 1.3312) (172.4343, 1.8702) knots 0 0 0 0 1 1 1 1
  spline S692 degree 3 poles (176.4841, 5.5492) (176.2735, 5.7527) (176.0628, 5.9562) (175.8521, 6.1597) knots 0 0 0 0 1 1 1 1
  spline S693 degree 3 poles (177.6814, 6.4104) (177.8088, 6.5235) (177.958, 6.6161) (178.0638, 6.7498) knots 0 0 0 0 1 1 1 1
  spline S694 degree 3 poles (178.0638, 6.7498) (178.1639, 6.8762) (178.2369, 7.0254) (178.2891, 7.178) knots 0 0 0 0 1 1 1 1
  spline S695 degree 3 poles (178.2891, 7.178) (178.3824, 7.451) (178.4279, 7.7381) (178.4973, 8.0181) knots 0 0 0 0 1 1 1 1
  spline S696 degree 3 poles (180.4965, 51.9621) (180.4886, 52.1069) (180.5719, 52.2908) (180.4726, 52.3965) knots 0 0 0 0 1 1 1 1
  spline S697 degree 3 poles (180.4726, 52.3965) (180.3178, 52.5616) (180.0544, 52.5696) (179.8453, 52.6562) knots 0 0 0 0 1 1 1 1
  spline S698 degree 3 poles (167.717, 165.3382) (167.2397, 165.2505) (166.7694, 165.1055) (166.285, 165.0749) knots 0 0 0 0 1 1 1 1
  spline S699 degree 3 poles (166.285, 165.0749) (165.1735, 165.0047) (164.0573, 165.0034) (162.9442, 165.0366) knots 0 0 0 0 1 1 1 1
  spline S700 degree 3 poles (162.9442, 165.0366) (162.3462, 165.0544) (161.7569, 165.1943) (161.1596, 165.2277) knots 0 0 0 0 1 1 1 1
  spline S701 degree 3 poles (161.1596, 165.2277) (160.711, 165.2527) (160.2601, 165.181) (159.8118, 165.2113) knots 0 0 0 0 1 1 1 1
  spline S702 degree 3 poles (159.8118, 165.2113) (159.3339, 165.2437) (158.8679, 165.396) (158.3893, 165.4155) knots 0 0 0 0 1 1 1 1
  spline S703 degree 3 poles (158.3893, 165.4155) (157.1155, 165.4674) (155.8393, 165.4532) (154.5647, 165.4252) knots 0 0 0 0 1 1 1 1
  spline S704 degree 3 poles (154.5647, 165.4252) (154.4123, 165.4219) (154.2608, 165.3781) (154.1191, 165.3218) knots 0 0 0 0 1 1 1 1
  spline S705 degree 3 poles (154.1191, 165.3218) (153.7811, 165.1874) (153.4289, 165.0664) (153.1323, 164.8557) knots 0 0 0 0 1 1 1 1
  spline S706 degree 3 poles (153.1323, 164.8557) (153.042, 164.7916) (153.0235, 164.6532) (153.0221, 164.5426) knots 0 0 0 0 1 1 1 1
  spline S707 degree 3 poles (153.0221, 164.5426) (152.9611, 159.9933) (153.0321, 155.4427) (152.9452, 150.8938) knots 0 0 0 0 1 1 1 1
  spline S708 degree 3 poles (152.9452, 150.8938) (152.9412, 150.6853) (152.7891, 150.5042) (152.7497, 150.2994) knots 0 0 0 0 1 1 1 1
  spline S709 degree 3 poles (152.7497, 150.2994) (152.7154, 150.1207) (152.7076, 149.9351) (152.7262, 149.7542) knots 0 0 0 0 1 1 1 1
  spline S710 degree 3 poles (152.7262, 149.7542) (152.7742, 149.2894) (152.9107, 148.836) (152.9488, 148.3703) knots 0 0 0 0 1 1 1 1
  spline S711 degree 3 poles (152.9488, 148.3703) (152.9859, 147.9171) (152.9892, 147.4593) (152.9512, 147.0062) knots 0 0 0 0 1 1 1 1
  spline S712 degree 3 poles (152.9512, 147.0062) (152.9214, 146.6501) (152.7848, 146.3091) (152.7465, 145.9538) knots 0 0 0 0 1 1 1 1
  spline S713 degree 3 poles (152.7465, 145.9538) (152.7098, 145.6129) (152.7271, 145.2683) (152.7272, 144.9255) knots 0 0 0 0 1 1 1 1
  spline S714 degree 3 poles (152.7272, 144.9255) (152.7274, 144.5828) (152.7058, 144.2377) (152.7474, 143.8974) knots 0 0 0 0 1 1 1 1
  spline S715 degree 3 poles (152.7474, 143.8974) (152.7839, 143.5999) (152.9377, 143.3225) (152.96, 143.0235) knots 0 0 0 0 1 1 1 1
  spline S716 degree 3 poles (152.96, 143.0235) (153.0108, 142.3432) (153.0101, 141.6576) (152.9654, 140.9767) knots 0 0 0 0 1 1 1 1
  spline S717 degree 3 poles (152.9654, 140.9767) (152.9343, 140.5011) (152.7385, 140.0423) (152.7333, 139.5656) knots 0 0 0 0 1 1 1 1
  spline S718 degree 3 poles (152.7333, 139.5656) (152.6718, 134.0224) (152.7435, 128.4785) (152.7653, 122.935) knots 0 0 0 0 1 1 1 1
  spline S719 degree 3 poles (152.7653, 122.935) (152.767, 122.5018) (152.7621, 122.0671) (152.8039, 121.6358) knots 0 0 0 0 1 1 1 1
  spline S720 degree 3 poles (152.8039, 121.6358) (152.8538, 121.121) (152.9613, 120.6134) (153.04, 120.1021) knots 0 0 0 0 1 1 1 1
  spline S721 degree 3 poles (152.7785, 117.5718) (152.8084, 117.0742) (152.8079, 116.5738) (152.8683, 116.079) knots 0 0 0 0 1 1 1 1
  spline S722 degree 3 poles (152.8683, 116.079) (152.903, 115.7944) (153.0377, 115.5267) (153.0629, 115.2411) knots 0 0 0 0 1 1 1 1
  spline S723 degree 3 poles (153.0629, 115.2411) (153.1052, 114.7629) (153.1056, 114.2796) (153.0696, 113.8009) knots 0 0 0 0 1 1 1 1
  spline S724 degree 3 poles (153.0696, 113.8009) (153.0336, 113.3234) (152.8455, 112.8605) (152.8477, 112.3818) knots 0 0 0 0 1 1 1 1
  spline S725 degree 3 poles (152.8477, 112.3818) (152.8499, 111.8943) (153.0589, 111.4253) (153.0827, 110.9385) knots 0 0 0 0 1 1 1 1
  spline S726 degree 3 poles (153.0827, 110.9385) (153.143, 109.7061) (153.1454, 108.4701) (153.0996, 107.2371) knots 0 0 0 0 1 1 1 1
  spline S727 degree 3 poles (153.0996, 107.2371) (153.0747, 106.567) (152.8803, 105.9088) (152.8708, 105.2383) knots 0 0 0 0 1 1 1 1
  spline S728 degree 3 poles (152.8708, 105.2383) (152.8163, 101.4245) (152.8266, 97.6091) (152.9077, 93.7958) knots 0 0 0 0 1 1 1 1
  spline S729 degree 3 poles (152.9077, 93.7958) (152.9224, 93.1025) (153.1336, 92.4236) (153.1579, 91.7306) knots 0 0 0 0 1 1 1 1
  spline S730 degree 3 poles (153.1579, 91.7306) (153.2285, 89.7135) (153.1055, 87.6922) (153.1918, 85.6757) knots 0 0 0 0 1 1 1 1
  spline S731 degree 3 poles (153.1918, 85.6757) (153.2087, 85.2821) (153.4026, 84.9148) (153.4662, 84.526) knots 0 0 0 0 1 1 1 1
  spline S732 degree 3 poles (153.4662, 84.526) (153.503, 84.3014) (153.49, 84.0713) (153.4917, 83.8437) knots 0 0 0 0 1 1 1 1
  spline S733 degree 3 poles (153.4917, 83.8437) (153.5102, 81.2801) (153.5232, 78.7164) (153.5268, 76.1528) knots 0 0 0 0 1 1 1 1
  spline S734 degree 3 poles (153.5268, 76.1528) (153.5295, 74.2027) (153.5658, 72.2518) (153.5105, 70.3024) knots 0 0 0 0 1 1 1 1
  spline S735 degree 3 poles (153.5105, 70.3024) (153.4979, 69.8593) (153.3363, 69.4288) (153.3235, 68.9857) knots 0 0 0 0 1 1 1 1
  spline S736 degree 3 poles (153.3235, 68.9857) (153.2866, 67.7054) (153.4078, 66.4235) (153.3617, 65.1435) knots 0 0 0 0 1 1 1 1
  spline S737 degree 3 poles (153.3617, 65.1435) (153.3469, 64.7339) (153.1492, 64.3436) (153.1416, 63.9339) knots 0 0 0 0 1 1 1 1
  spline S738 degree 3 poles (153.1416, 63.9339) (153.0775, 60.5123) (153.117, 57.0894) (153.1468, 53.6673) knots 0 0 0 0 1 1 1 1
  spline S739 degree 3 poles (153.1468, 53.6673) (153.1523, 53.037) (153.2388, 52.4092) (153.2474, 51.779) knots 0 0 0 0 1 1 1 1
  spline S740 degree 3 poles (153.2474, 51.779) (153.2539, 51.3007) (153.244, 50.8205) (153.1921, 50.345) knots 0 0 0 0 1 1 1 1
  spline S741 degree 3 poles (153.1921, 50.345) (153.1805, 50.2388) (153.0527, 50.1599) (153.0591, 50.0532) knots 0 0 0 0 1 1 1 1
  spline S742 degree 3 poles (153.0591, 50.0532) (153.0666, 49.9287) (153.1954, 49.8399) (153.2297, 49.7199) knots 0 0 0 0 1 1 1 1
  spline S743 degree 3 poles (153.2297, 49.7199) (153.3431, 49.322) (153.4096, 48.9121) (153.4996, 48.5082) knots 0 0 0 0 1 1 1 1
  spline S744 degree 3 poles (153.1918, 85.6757) (153.1191, 85.0968) (152.9817, 84.5224) (152.9738, 83.9391) knots 0 0 0 0 1 1 1 1
  spline S745 degree 3 poles (152.9738, 83.9391) (152.922, 80.0981) (152.9874, 76.2564) (153.013, 72.4151) knots 0 0 0 0 1 1 1 1
  spline S746 degree 3 poles (153.013, 72.4151) (153.0179, 71.6693) (152.9982, 70.921) (153.0654, 70.1782) knots 0 0 0 0 1 1 1 1
  spline S747 degree 3 poles (153.0654, 70.1782) (153.1021, 69.7731) (153.2375, 69.3832) (153.3235, 68.9857) knots 0 0 0 0 1 1 1 1
  spline S748 degree 3 poles (153.0591, 50.0532) (152.8615, 50.0991) (152.6638, 50.1449) (152.4661, 50.1907) knots 0 0 0 0 1 1 1 1
  spline S749 degree 3 poles (153.3617, 65.1435) (153.4388, 64.933) (153.5461, 64.7313) (153.593, 64.5121) knots 0 0 0 0 1 1 1 1
  spline S750 degree 3 poles (153.593, 64.5121) (153.6335, 64.3231) (153.6189, 64.1262) (153.621, 63.9329) knots 0 0 0 0 1 1 1 1
  spline S751 degree 3 poles (153.621, 63.9329) (153.6728, 59.2392) (153.7918, 54.5454) (153.7549, 49.8516) knots 0 0 0 0 1 1 1 1
  spline S752 degree 3 poles (153.7549, 49.8516) (153.7513, 49.3958) (153.5536, 48.9608) (153.4996, 48.5082) knots 0 0 0 0 1 1 1 1
  spline S753 degree 3 poles (153.4996, 48.5082) (153.4036, 47.7026) (153.3213, 46.8932) (153.3054, 46.0821) knots 0 0 0 0 1 1 1 1
  spline S754 degree 3 poles (153.3054, 46.0821) (153.2551, 43.5174) (153.2948, 40.9518) (153.3012, 38.3867) knots 0 0 0 0 1 1 1 1
  spline S755 degree 3 poles (153.3012, 38.3867) (153.3017, 38.195) (153.2938, 38.001) (153.3262, 37.8121) knots 0 0 0 0 1 1 1 1
  spline S756 degree 3 poles (153.3262, 37.8121) (153.3779, 37.5102) (153.477, 37.2184) (153.5524, 36.9215) knots 0 0 0 0 1 1 1 1
  spline S757 degree 3 poles (153.5028, 47.9018) (153.5722, 47.6643) (153.665, 47.4324) (153.7108, 47.1892) knots 0 0 0 0 1 1 1 1
  spline S758 degree 3 poles (153.7108, 47.1892) (153.748, 46.9916) (153.749, 46.7882) (153.7507, 46.5871) knots 0 0 0 0 1 1 1 1
  spline S759 degree 3 poles (153.7507, 46.5871) (153.7712, 44.0481) (153.7873, 41.509) (153.7772, 38.9699) knots 0 0 0 0 1 1 1 1
  spline S760 degree 3 poles (153.7772, 38.9699) (153.7754, 38.5143) (153.7648, 38.0574) (153.7151, 37.6045) knots 0 0 0 0 1 1 1 1
  spline S761 degree 3 poles (153.7151, 37.6045) (153.6896, 37.3719) (153.5835, 37.1535) (153.5524, 36.9215) knots 0 0 0 0 1 1 1 1
  spline S762 degree 3 poles (153.5524, 36.9215) (153.4732, 36.3294) (153.4125, 35.734) (153.3847, 35.1372) knots 0 0 0 0 1 1 1 1
  spline S763 degree 3 poles (153.3847, 35.1372) (153.3342, 34.0526) (153.3123, 32.9663) (153.3177, 31.8805) knots 0 0 0 0 1 1 1 1
  spline S764 degree 3 poles (153.3177, 31.8805) (153.3258, 30.2179) (153.3306, 28.5537) (153.4251, 26.8937) knots 0 0 0 0 1 1 1 1
  spline S765 degree 3 poles (153.4251, 26.8937) (153.4518, 26.4253) (153.5953, 25.9709) (153.6804, 25.5095) knots 0 0 0 0 1 1 1 1
  spline S766 degree 3 poles (153.6934, 24.217) (153.6362, 23.5681) (153.5283, 22.9217) (153.5218, 22.2704) knots 0 0 0 0 1 1 1 1
  spline S767 degree 3 poles (153.5218, 22.2704) (153.4952, 19.581) (153.502, 16.89) (153.5941, 14.202) knots 0 0 0 0 1 1 1 1
  spline S768 degree 3 poles (153.5941, 14.202) (153.6098, 13.7446) (153.4282, 12.6624) (153.8447, 12.8521) knots 0 0 0 0 1 1 1 1
  spline S769 degree 3 poles (153.8447, 12.8521) (154.3152, 13.0663) (154.0068, 13.8767) (154.0149, 14.3936) knots 0 0 0 0 1 1 1 1
  spline S770 degree 3 poles (154.0149, 14.3936) (154.0546, 16.9342) (154.0708, 19.4766) (153.9877, 22.0161) knots 0 0 0 0 1 1 1 1
  spline S771 degree 3 poles (153.9877, 22.0161) (153.9635, 22.7559) (153.7582, 23.4797) (153.6934, 24.217) knots 0 0 0 0 1 1 1 1
  spline S772 degree 3 poles (153.6934, 24.217) (153.6556, 24.6462) (153.6482, 25.0799) (153.6804, 25.5095) knots 0 0 0 0 1 1 1 1
  spline S773 degree 3 poles (153.6804, 25.5095) (153.7177, 26.0068) (153.8823, 26.4909) (153.9013, 26.9893) knots 0 0 0 0 1 1 1 1
  spline S774 degree 3 poles (153.9013, 26.9893) (153.9501, 28.2707) (153.9352, 29.555) (153.8835, 30.8364) knots 0 0 0 0 1 1 1 1
  spline S775 degree 3 poles (153.8835, 30.8364) (153.8676, 31.2324) (153.7011, 31.6146) (153.6988, 32.0109) knots 0 0 0 0 1 1 1 1
  spline S776 degree 3 poles (153.6988, 32.0109) (153.6971, 32.2798) (153.8505, 32.5308) (153.8717, 32.7989) knots 0 0 0 0 1 1 1 1
  spline S777 degree 3 poles (153.8717, 32.7989) (153.92, 33.408) (153.9017, 34.0207) (153.9063, 34.6317) knots 0 0 0 0 1 1 1 1
  spline S778 degree 3 poles (153.9063, 34.6317) (153.9077, 34.8109) (153.9192, 34.9923) (153.8896, 35.169) knots 0 0 0 0 1 1 1 1
  spline S779 degree 3 poles (153.8896, 35.169) (153.8013, 35.6963) (153.6655, 36.2145) (153.5535, 36.7372) knots 0 0 0 0 1 1 1 1